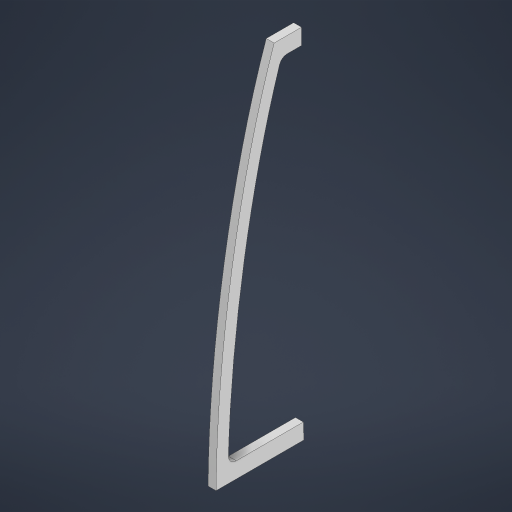
# Autodesk Inventor part: nose_spanner
Saved by Autodesk Inventor 2023 (Build 270158030, 158C)
## iProperties
Created: 2022-07-02
Part Number: nose_spanner
Material: Generic
Document SubType Name: Modeling
Designer: kardo
Density: 1 g/cm^3
Appearance: Default
Author: kardo
Autodesk Inventor part; units mm, degrees
ref_plane "YZ Plane" through (0, 0, 0) normal (1, 0, 0) x (0, 1, 0)
ref_plane "XZ Plane" through (0, 0, 0) normal (0, 1, 0) x (-1, 0, 0)
ref_plane "XY Plane" through (0, 0, 0) normal (0, 0, 1) x (1, 0, 0)
derived "surface_body.ipt"
sketch "sk_rail_top_tunnel" plane through (81.12, 0, 0) normal (1, 0, 0) x (0, 1, 0)
  line L0 (237, 107.6209) -> (237, -224.5198)
  line L1 (0, 107.6209) -> (0, -224.5198)
  line L2 (-363, 107.6209) -> (-363, -224.5198)
  line L3 (-363, 0) -> (0, 0)
  line L4 (-181.5, 48.8998) -> (-181.5, 0)
  line L5 (0, 52.89) -> (31.284, 52.89)
  line L6 (31.284, 52.89) -> (68.256, 47.0555)
  line L7 (68.256, 47.0555) -> (94.8, 37.536)
  line L8 (94.8, 107.6209) -> (94.8, -224.5198)
  line L9 (0, 52.89) -> (237, 52.89)
  line L10 (-488.1035, 0) -> (361.1125, 0)
  spline S0 degree 3 poles (0, 52.89) (86.3106, 52.89) (181.3207, 49.5034) (237, 36.448) knots 0 0 0 0 1 1 1 1
  spline S1 degree 3 poles (0, 52.89) (31.284, 52.89) (68.256, 47.0555) (94.8, 37.536) knots 1 1 1 1 2 2 2 2
  spline S2 degree 4 poles (-363, 37.4293) (-272.3626, 45.1427) (-181.5879, 49.7528) (-90.8131, 52.89) (0, 52.89) knots 0 0 0 0 0 1 1 1 1 1
  point P0 (142.2, 48.7795)
  point P1 (94.8, 28.832)
  point P2 (-242.0001, 45.8501)
  point P3 (-120.9999, 51.0063)
sketch "sk_rail_bottom_tunnel" plane through (81.12, 0, 0) normal (1, 0, 0) x (0, 1, 0)
  line L0 (-254.1001, 19.9549) -> (9.48, 28.4869)
  arc A0 (30.81, 28.832) -> (9.48, 28.4869) centre (30.81, -630.4631) ccw
  line L1 (30.81, 28.832) -> (94.8, 28.832)
  arc A1 (-275.8801, 19.4795) -> (-254.1001, 19.9549) centre (-287.5515, 1053.3708) ccw
  line L2 (-363, 18.496) -> (-275.8801, 19.4795)
  point P0 (0, 0)
ref_plane "plane_tunnel_right" through (81.12, 0, 0) normal (1, 0, 0) x (0, 1, 0)
ref_plane "plane_middle" through (0, 0, 0) normal (0, 1, 0) x (-1, 0, 0)
derived "parameters_frame.ipt"
sketch "sk_base" plane through (81.12, 0, 0) normal (1, 0, 0) x (0, 1, 0)
  spline S0 degree 3 poles (0, 52.89) (31.284, 52.89) (68.256, 47.0555) (94.8, 37.536) knots 1 1 1 1 2 2 2 2 construction
  line L0 (30.81, 28.832) -> (94.8, 28.832) construction
  arc A0 (30.81, 28.832) -> (9.48, 28.4869) centre (30.81, -630.4631) ccw construction
  line L1 (-254.1001, 19.9549) -> (9.48, 28.4869) construction
  line L2 (0, 1390.1376) -> (0, -967.2299) construction
  line L3 (92.8, 36.9696) -> (92.8, 30.032)
  line L4 (92.8, 30.032) -> (88.8, 30.032)
  line L5 (88.8, 35.1542) -> (88.8, 30.032)
  line L6 (92.8, 30.032) -> (92.8, 28.832) construction
  line L7 (94.8, 37.536) -> (94.8, 28.832) construction
  line L8 (2, 51.6821) -> (2, 29.4454)
  line L9 (2, 29.4454) -> (6, 29.5748)
  line L10 (6, 29.5748) -> (6, 48.6194)
  line L11 (6, 29.5748) -> (6.0388, 28.3755)
  line L12 (2, 29.4454) -> (2.0388, 28.246)
  spline S1 degree 5 poles (2, 51.682) (11.4414, 51.6077) (20.8786, 51.1028) (30.2896, 50.2612) (48.6295, 47.9834) (66.765, 44.4259) (75.5596, 42.3591) (84.2725, 39.9338) (92.8, 36.9695) knots 0 0 0 0 0 0 0.511201 0.511201 0.511201 1 1 1 1 1 1
  spline S2 degree 5 poles (6, 48.6194) (14.5435, 48.4213) (23.079, 47.8852) (31.5914, 47.0728) (48.2972, 44.9453) (64.8318, 41.7452) (72.9132, 39.892) (80.927, 37.7381) (88.8, 35.1541) knots 0 0 0 0 0 0 0.507709 0.507709 0.507709 1 1 1 1 1 1
  point P0 (0, 0)
  dimension "d3" = 4.2
  dimension "d11" = 1.2
  dimension "d5" = 4
  dimension "d6" = 1.2
  dimension "d7" = 2
  dimension "d8" = 2
  dimension "d9" = 4
  dimension "d10" = 1.2
  constraints: 20 end point, 6 parallel, 3 perpendicular, 3 point on line, 6 other
  measures "d5" distance between parallel lines of L3 L5
  measures "d6" distance of L3.end L6.end
  measures "d7" distance between parallel lines of L7 L3
  measures "d8" distance between parallel lines of L2 L8
  measures "d9" distance between parallel lines of L8 L10
  measures "d10" distance of L9.end L11.end
extrude "Extrusion1" add sketch "sk_base" against normal blind 2
fillet "Fillet1" radius 2 2 edges at (80.12, 88.8, 35.1541) (80.12, 6, 48.6194)
equation "\"d3\" = shell_thickness + 0.75 * bulkhead_inset"
equation "\"d11\" = shell_thickness"
equation "\"d5\" = bulkhead_inset"
equation "\"d6\" = shell_thickness"
equation "\"d7\" = bulkhead_thickness"
equation "\"d8\" = bulkhead_thickness"
equation "\"d9\" = bulkhead_inset"
equation "\"d10\" = shell_thickness"
equation "\"d12\" = bulkhead_thickness"
equation "\"d14\" = 0.5 * bulkhead_inset"
equation "\"shell_thickness\" = 1.2"
equation "\"bulkhead_inset\" = 4"
equation "\"bulkhead_thickness\" = 2"
body "Solid1"
